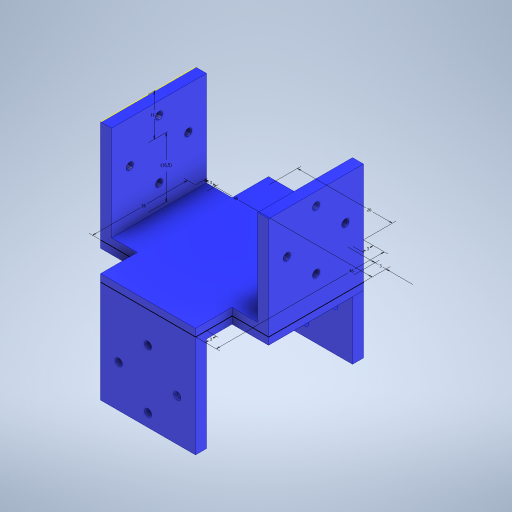
# Autodesk Inventor part: first_junction
Saved by Autodesk Inventor 2024 (Build 280153000, 153)
## iProperties
Created: 2024-02-16
Part Number: first_junction
Material: Generic
Document SubType Name: Modeling
Designer: kamil
Density: 1 g/cm^3
Appearance: Blue - Wall Paint - Glossy
Author: kamil
Autodesk Inventor part; units mm, degrees
ref_plane "YZ Plane" through (0, 0, 0) normal (1, 0, 0) x (0, 1, 0)
ref_plane "XZ Plane" through (0, 0, 0) normal (0, 1, 0) x (-1, 0, 0)
ref_plane "XY Plane" through (0, 0, 0) normal (0, 0, 1) x (1, 0, 0)
sketch "Sketch1" plane through (0, 0, 0) normal (0, 1, 0) x (-1, 0, 0)
  line L0 (23, 13) -> (-23, 13)
  line L1 (-23, 13) -> (-23, -13)
  line L2 (-23, -13) -> (23, -13)
  line L3 (23, -13) -> (23, 13)
  line L4 (13, 23) -> (-13, 23)
  line L5 (-13, 23) -> (-13, -23)
  line L6 (-13, -23) -> (13, -23)
  line L7 (13, -23) -> (13, 23)
  line L8 (13, -23) -> (-13, 23) construction
  line L9 (13, 23) -> (-13, -23) construction
  line L10 (23, -13) -> (-23, 13) construction
  line L11 (23, 13) -> (-23, -13) construction
  line L12 (13, -23) -> (-13, -23)
  line L13 (-13, -23) -> (-13, -20)
  line L14 (-13, -20) -> (13, -20)
  line L15 (13, -20) -> (13, -23)
  line L16 (13, 23) -> (-13, 23)
  line L17 (-13, 23) -> (-13, 20)
  line L18 (-13, 20) -> (13, 20)
  line L19 (13, 20) -> (13, 23)
  line L20 (23, 13) -> (20, 13)
  line L21 (20, 13) -> (20, -13)
  line L22 (20, -13) -> (23, -13)
  line L23 (23, -13) -> (23, 13)
  line L24 (-23, 13) -> (-20, 13)
  line L25 (-20, 13) -> (-20, -13)
  line L26 (-20, -13) -> (-23, -13)
  line L27 (-23, -13) -> (-23, 13)
  point P0 (0, 0)
  point P1 (0, 0)
  point P2 (0, 0)
  point P3 (13, 20)
  point P4 (13, 13)
  point P5 (-13, 13)
  point P6 (-13, -13)
  point P7 (13, -13)
  dimension "d0" = 46
  dimension "d1" = 46
  dimension "d2" = 26
  dimension "d3" = 26
  dimension "d4" = 3
  dimension "d5" = 3
  dimension "d6" = 3
  dimension "d7" = 3
  constraints: 56 end point, 12 parallel, 6 horizontal, 6 perpendicular, 4 point on line, 3 midpoint, 1 coincident
  measures "d0" distance of L1.end L2.end
  measures "d1" distance of L4.end L5.end
  measures "d2" distance between parallel lines of L2 L0
  measures "d3" distance between parallel lines of L5 L7
  measures "d4" distance of L12.end L13.end
  measures "d5" distance of L17.end L16.end
  measures "d6" distance of L22.end L21.end
  measures "d7" distance of L25.end L26.end
extrude "Extrusion1" add sketch "Sketch1" along normal blind 28 contours L3 L2 L21 L0 | L25 L2 L1 L0
extrude "Extrusion2" add sketch "Sketch1" against normal blind 28 contours L18 L5 L4 L7 | L7 L6 L5 L14
extrude "Extrusion3" add sketch "Sketch1" along normal mid plane 4 contours L21 L2 L7 L0 | L7 L2 L5 L0 | L0 L5 L18 L7 | L5 L2 L25 L0 | L7 L14 L5 L2
extrude "Extrusion4" add sketch "Sketch1" along normal blind 2 contours L18 L5 L4 L7 | L7 L6 L5 L14
extrude "Extrusion5" add sketch "Sketch1" against normal blind 2 contours L3 L2 L21 L0 | L25 L2 L1 L0
sketch "Sketch2" plane through (23, 28, 13) normal (1, 0, 0) x (0, 0, -1)
  line L0 (0, 0) -> (26, 0) projected
  line L1 (13, 0) -> (13, -11.5)
  circle A0 centre (13, -19.5) radius 1
  circle A1 centre (21, -11.5) radius 1
  circle A2 centre (13, -3.5) radius 1
  circle A3 centre (5, -11.5) radius 1
  point P0 (13, -28)
  dimension "d18" = 11.5
  dimension "d19" = 2
  dimension "d20" = 8
  dimension "d24" = 360
  constraints: 4 centre point, 2 end point, 1 midpoint, 1 vertical, 9 other
  measures "d18" distance of L1.start L1.end
  measures "d19" diameter of A0
  measures "d20" distance of A0.centre L1.end
extrude "Extrusion6" cut sketch "Sketch2" against normal blind 60
sketch "Sketch3" plane through (-13, -28, 23) normal (0, 0, 1) x (1, 0, 0)
  line L0 (0, 0) -> (26, 0) projected
  line L1 (13, 0) -> (13, 11.5)
  circle A0 centre (13, 19.5) radius 1
  circle A1 centre (5, 11.5) radius 1
  circle A2 centre (13, 3.5) radius 1
  circle A3 centre (21, 11.5) radius 1
  point P0 (13, 28)
  dimension "d28" = 11.5
  dimension "d29" = 2
  dimension "d30" = 8
  dimension "d33" = 360
  constraints: 4 centre point, 2 end point, 1 midpoint, 1 vertical, 9 other
  measures "d28" distance of L1.start L1.end
  measures "d29" diameter of A0
  measures "d30" distance of L1.end A0.centre
extrude "Extrusion7" cut sketch "Sketch3" against normal blind 60
sketch "Sketch4" plane through (-23, 28, -13) normal (-1, 0, 0) x (0, 0, 1)
  line L0 (0, 0) -> (26, 0) projected
  line L1 (13, 0) -> (13, -11.5)
  point P0 (13, -28)
  dimension "d37" = 11.5
  dimension "d38" = 16.5
  constraints: 2 end point, 1 midpoint, 1 vertical
  measures "d37" distance of L1.start L1.end
  measures "d38" distance of point (13, -28) L1.end
body "Solid1"
